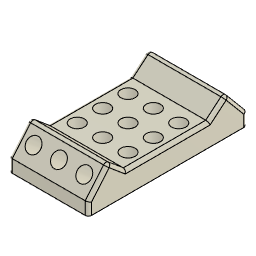
Heat Set Insert Practice Block (Autodesk Fusion 360 design; units mm, degrees)
Autodesk Fusion 360 part; units mm, degrees
sketch "Outline" plane through (0, 0, 0) normal (0, 0, 1) x (1, 0, 0)
  line L0 (12.5, -25) -> (-12.5, -25)
  line L1 (-12.5, -25) -> (-12.5, 25)
  line L2 (-12.5, 25) -> (12.5, 25)
  line L3 (12.5, 25) -> (12.5, -25)
  line L4 (12.5, -25) -> (-12.5, 25) construction
  line L5 (-12.5, -25) -> (12.5, 25) construction
  dimension "d1" = 25
  dimension "d2" = 50
  constraint horizontal L0
  constraint perpendicular L0 L1
  constraint parallel L0 L2
  constraint parallel L1 L3
  constraint coincident L4 origin
  constraint coincident L5 origin
  measures "d1" distance of L1.end L2.end
  measures "d2" distance of L0.end L1.end
extrude "Extrude1" add sketch "Outline" along normal blind 7
sketch "50 Degree Angle" plane through (12.5, 0, 0) normal (1, 0, 0) x (0, 1, 0)
  line L0 (-25, 0) -> (25, 0)
  line L1 (25, 0) -> (25, 7)
  line L2 (25, 7) -> (-25, 7)
  line L3 (-25, 7) -> (-25, 0)
  line L4 (-25, 0) -> (-25, 4)
  line L5 (-25, 4) -> (-18.5721, 11.6604)
  line L6 (-25, 4) -> (-15, 4) construction
  line L7 (-18.5721, 11.6604) -> (-13.018, 7)
  line L8 (0, 7) -> (0, 13) construction
  line L9 (25, 0) -> (25, 4)
  line L10 (25, 4) -> (18.5721, 11.6604)
  line L11 (18.5721, 11.6604) -> (13.018, 7)
  dimension "d5" = 4
  dimension "d6" = 50
  dimension "d7" = 10
  constraint coincident L0.start L3.end
  constraint perpendicular L0 L4
  constraint horizontal L6
  constraint coincident L2 L7.end
  constraint perpendicular L5 L7
  constraint midpoint L2 L8.start
  constraint perpendicular L2 L8
  constraint symmetric L0.start L8 L0.end
  constraint symmetric L4.end L8 L9.end
  constraint symmetric L5.end L8 L10.end
  constraint symmetric L7.end L8 L11.end
  measures "d5" distance of L0.start L4.end
  measures "d6" angle of L5 L6
  measures "d7" distance of L4.end L5.end
extrude "Extrude2" cut sketch "50 Degree Angle" against normal blind 25 contours L2 L3 L5 | L1 L2 L10
extrude "Extrude3" add sketch "50 Degree Angle" against normal blind 25 contours L2 L5 L7 | L2 L10 L11
sketch "Side 1 Holes" plane through (0, -16.6402, 13.9628) normal (0, -0.766044, 0.642788) x (1, 0, 0)
  line L0 (12.5, -13.0055) -> (12.5, -3.0055)
  line L1 (12.5, -3.0055) -> (-12.5, -3.0055)
  line L2 (-12.5, -3.0055) -> (-12.5, -13.0055)
  line L3 (-12.5, -13.0055) -> (12.5, -13.0055)
  line L4 (-12.5, -8.0055) -> (12.5, -8.0055) construction
  circle A0 centre (0, -8.0055) radius 2.25
  circle A1 centre (-8, -8.0055) radius 2.25
  circle A2 centre (8, -8.0055) radius 2.25
  dimension "d12" = 4.5
  dimension "d15" = 8
  dimension "d16" = 0
  constraint midpoint L2 L4.start
  constraint midpoint L0 L4.end
  constraint midpoint L4 A0.centre
  measures "d12" diameter of A0
sketch "Side 2 Holes" plane through (0, 16.6402, 13.9628) normal (0, 0.766044, 0.642788) x (-1, 0, 0)
  line L0 (-12.5, -3.0055) -> (-12.5, -13.0055)
  line L1 (-12.5, -13.0055) -> (12.5, -13.0055)
  line L2 (12.5, -13.0055) -> (12.5, -3.0055)
  line L3 (12.5, -3.0055) -> (-12.5, -3.0055)
  line L4 (-12.5, -8.0055) -> (12.5, -8.0055) construction
  circle A0 centre (0, -8.0055) radius 2.25
  circle A1 centre (-8, -8.0055) radius 2.25
  circle A2 centre (8, -8.0055) radius 2.25
  dimension "d17" = 4.5
  dimension "d20" = 8
  dimension "d21" = 0
  constraint midpoint L0 L4.start
  constraint midpoint L2 L4.end
  constraint midpoint L4 A0.centre
  measures "d17" diameter of A0
sketch "Top Holes" plane through (0, 0, 7) normal (0, 0, 1) x (-1, 0, 0)
  line L0 (-12.5, -13.018) -> (12.5, -13.018)
  line L1 (12.5, -13.018) -> (12.5, 13.018)
  line L2 (12.5, 13.018) -> (-12.5, 13.018)
  line L3 (-12.5, 13.018) -> (-12.5, -13.018)
  circle A0 centre (0, 0) radius 2.25
  circle A1 centre (-8, -8) radius 2.25
  circle A2 centre (0, -8) radius 2.25
  circle A3 centre (8, -8) radius 2.25
  circle A4 centre (-8, 0) radius 2.25
  circle A5 centre (8, 0) radius 2.25
  circle A6 centre (-8, 8) radius 2.25
  circle A7 centre (0, 8) radius 2.25
  circle A8 centre (8, 8) radius 2.25
  dimension "d22" = 4.5
  dimension "d25" = 8
  dimension "d26" = 8
  constraint coincident A0.centre origin
  measures "d22" diameter of A0
extrude "Extrude4" cut sketch "Side 1 Holes" against normal blind 6 draft -4 contours A0 | A1 | A2
extrude "Extrude5" cut sketch "Top Holes" against normal blind 6 draft -4 contours A0 | A1 | A2 | A3 | A4 | A5 | A6 | A7 | A8
extrude "Extrude6" cut sketch "Side 2 Holes" against normal blind 6 draft -4 contours A0 | A1 | A2
extrude "Extrude7" cut 3 faces at (7.8243, 16.923, 4.2914) (0.4373, 17.0087, 4.1893) (-8.2782, 17.0196, 4.1763) along direction (0, 0.766044, 0.642788) up to surface end surface through (0, 0, 0) normal (0, 0, -1) offset 0
extrude "Extrude8" cut 3 faces at (8.6033, -17.3625, 3.7676) (-0.5009, -17.3448, 3.7887) (-8.144, -17.8914, 3.1373) along direction (0, -0.766044, 0.642788) up to surface end surface through (0, 0, 0) normal (0, 0, -1) offset 0
extrude "Extrude9" cut 9 faces at (7.3634, -7.6464, 1) (7.4373, 0.0909, 1) (7.4373, 8.0909, 1) (-0.7188, 8.415, 1) (-8.4961, 8.0909, 1) (-8.4806, 0.4999, 1) (0.57, -0.3536, 1) (-8.5009, -7.4112, 1) (-0.7188, -7.585, 1) along direction (0, 0, 1) up to surface end surface through (0, 0, 0) normal (0, 0, -1) offset 0
fillet "Fillet1" radius 1 2 edges at (0, -18.5721, 11.6604) (0, 18.5721, 11.6604)
fillet "Fillet2" radius 1 18 edges at (12.5, -15.4121, 9.0088) (12.5, -18.536, 11.2478) (12.5, -22.1075, 7.4472) (12.5, -25, 2) (12.5, 0, 7) (12.5, 22.1075, 7.4472) (12.5, 18.536, 11.2478) (12.5, 15.4121, 9.0088) (12.5, 25, 2) (-12.5, 25, 2) (-12.5, 15.4121, 9.0088) (-12.5, 18.536, 11.2478) (-12.5, 22.1075, 7.4472) (-12.5, 0, 7) (-12.5, -22.1075, 7.4472) (-12.5, -18.536, 11.2478) (-12.5, -15.4121, 9.0088) (-12.5, -25, 2)
